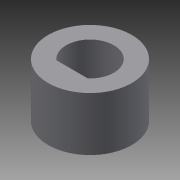
# Autodesk Inventor part: newStepperCollar
Saved by Autodesk Inventor 2013 SP2 (Build 170200200, 200)
## iProperties
Created: 2016-05-16
Part Number: newStepperCollar
Material: Generic
Document SubType Name: Modeling
Designer: 2016ahoganso
Density: 1 g/cm^3
Author: 2016ahoganso
Autodesk Inventor part; units mm, degrees
ref_plane "YZ Plane" through (0, 0, 0) normal (1, 0, 0) x (0, 1, 0)
ref_plane "XZ Plane" through (0, 0, 0) normal (0, 1, 0) x (-1, 0, 0)
ref_plane "XY Plane" through (0, 0, 0) normal (0, 0, 1) x (1, 0, 0)
sketch "Sketch1" plane through (0, 0, 0) normal (0, 1, 0) x (-1, 0, 0)
  arc A0 (-2.6458, 3) -> (2.6458, 3) centre (0, 0) ccw
  line L0 (-2.6458, 3) -> (2.6458, 3)
  circle A1 centre (0, 0) radius 7
  dimension "d5" = 14
  constraints: 2 centre point, 2 coincident, 2 end point, 2 point on circle
  measures "d5" diameter of A1
extrude "Extrusion1" add sketch "Sketch1" along normal blind 9
body "Solid1"
